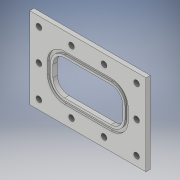
# Autodesk Inventor part: Front
Saved by Autodesk Inventor 2018.1 (Build 221171000, 171)
## iProperties
Created: 2018-04-18
Part Number: Front
Material: Generic
Document SubType Name: Modeling
Designer: trent
Density: 1 g/cm^3
Appearance: Default
Author: trent
Autodesk Inventor part; units mm, degrees
ref_plane "YZ Plane" through (0, 0, 0) normal (1, 0, 0) x (0, 1, 0)
ref_plane "XZ Plane" through (0, 0, 0) normal (0, 1, 0) x (-1, 0, 0)
ref_plane "XY Plane" through (0, 0, 0) normal (0, 0, 1) x (1, 0, 0)
sketch "Sketch1" plane through (0, 0, 0) normal (0, 0, 1) x (1, 0, 0)
  line L0 (0, 0) -> (127, 0)
  line L1 (127, 0) -> (127, 88.9)
  line L2 (127, 88.9) -> (0, 88.9)
  line L3 (0, 88.9) -> (0, 0)
  circle A0 centre (10.16, 78.74) radius 3.0988
  circle A1 centre (10.16, 44.45) radius 3.0988
  circle A2 centre (10.16, 10.16) radius 3.0988
  circle A3 centre (45.72, 10.16) radius 3.0988
  circle A4 centre (116.84, 10.16) radius 3.0988
  circle A5 centre (116.84, 44.45) radius 3.0988
  circle A6 centre (116.84, 78.74) radius 3.0988
  circle A7 centre (45.72, 78.74) radius 3.0988
  line L4 (25.4, 25.4) -> (101.6, 25.4)
  line L5 (101.6, 25.4) -> (101.6, 63.5)
  line L6 (101.6, 63.5) -> (25.4, 63.5)
  line L7 (25.4, 63.5) -> (25.4, 25.4)
  line L8 (25.4, 25.4) -> (101.6, 63.5) construction
  line L9 (101.6, 25.4) -> (25.4, 63.5) construction
  circle A8 centre (81.28, 10.16) radius 3.0988
  circle A9 centre (81.28, 78.74) radius 3.0988
  point P0 (63.5, 44.45)
  dimension "d0" = 127
  dimension "d1" = 88.9
  dimension "d3" = 6.1976
  dimension "d4" = 10.16
  dimension "d5" = 10.16
  dimension "d6" = 10.16
  dimension "d7" = 10.16
  dimension "d8" = 44.45
  dimension "d10" = 10.16
  dimension "d11" = 10.16
  dimension "d12" = 10.16
  dimension "d13" = 10.16
  dimension "d14" = 44.45
  dimension "d15" = 10.16
  dimension "d16" = 10.16
  dimension "d17" = 10.16
  dimension "d18" = 10.16
  dimension "d31" = 76.2
  dimension "d32" = 38.1
  dimension "d33" = 44.45
  dimension "d34" = 63.5
  dimension "d42" = 35.56
  dimension "d43" = 35.56
  dimension "d44" = 35.56
  dimension "d46" = 35.56
  dimension "d47" = 35.56
  dimension "d49" = 35.56
  constraints: 20 end point, 10 centre point, 9 equal radius, 4 parallel, 2 horizontal, 2 midpoint, 2 perpendicular
  measures "d0" distance of L2.end L1.end
  measures "d1" distance of L1.end L0.end
  measures "d3" diameter of A0
  measures "d4" distance from line of L2 A0.centre
  measures "d5" distance from line of L3 A0.centre
  measures "d6" distance from line of L3 A2.centre
  measures "d7" distance from line of L0 A2.centre
  measures "d8" distance from line of L0 A1.centre
  measures "d10" distance from line of L2 A7.centre
  measures "d11" distance from line of L3 A1.centre
  measures "d12" distance from line of L2 A6.centre
  measures "d13" distance from line of L1 A6.centre
  measures "d14" distance from line of L0 A5.centre
  measures "d15" distance from line of L1 A5.centre
  measures "d16" distance from line of L0 A4.centre
  measures "d17" distance from line of L1 A4.centre
  measures "d18" distance from line of L0 A3.centre
  measures "d31" distance of L6.end L5.end
  measures "d32" distance of L5.end L4.end
  measures "d33" distance from line of L0 point (63.5, 44.45)
  measures "d34" distance from line of L1 point (63.5, 44.45)
  measures "d42" distance of A0.centre A7.centre
  measures "d43" distance of A7.centre A9.centre
  measures "d44" distance of A6.centre A9.centre
  measures "d46" distance of A8.centre A3.centre
  measures "d47" distance of A2.centre A3.centre
  measures "d49" distance of A4.centre A8.centre
extrude "Extrusion1" add sketch "Sketch1" along normal blind 4.7625
thread "Thread1" size "M6x1" class "6H" standard "ANSI Metric M Profile" full length
thread "Thread2" size "M6x1" class "6H" standard "ANSI Metric M Profile" full length
thread "Thread3" size "M6x1" class "6H" standard "ANSI Metric M Profile" full length
thread "Thread4" size "M6x1" class "6H" standard "ANSI Metric M Profile" full length
thread "Thread5" size "M6x1" class "6H" standard "ANSI Metric M Profile" full length
thread "Thread6" size "M6x1" class "6H" standard "ANSI Metric M Profile" full length
thread "Thread7" size "M6x1" class "6H" standard "ANSI Metric M Profile" full length
thread "Thread8" size "M6x1" class "6H" standard "ANSI Metric M Profile" full length
thread "Thread9" size "M6x1" class "6H" standard "ANSI Metric M Profile" full length
fillet "Fillet3" radius 12.7 4 edges at (101.6, 63.5, 2.3813) (101.6, 25.4, 2.3813) (25.4, 63.5, 2.3813) (25.4, 25.4, 2.3813)
sketch "Sketch4" plane through (0, 0, 4.7625) normal (0, 0, 1) x (1, 0, 0)
  arc A0 (38.1, 63.5) -> (25.4, 50.8) centre (38.1, 50.8) ccw projected
  arc A1 (38.1, 63.5) -> (25.4, 50.8) centre (38.1, 50.8) ccw
  arc A2 (101.6, 50.8) -> (88.9, 63.5) centre (88.9, 50.8) ccw projected
  arc A3 (101.6, 50.8) -> (88.9, 63.5) centre (88.9, 50.8) ccw
  arc A4 (88.9, 25.4) -> (101.6, 38.1) centre (88.9, 38.1) ccw projected
  arc A5 (88.9, 25.4) -> (101.6, 38.1) centre (88.9, 38.1) ccw
  arc A6 (25.4, 38.1) -> (38.1, 25.4) centre (38.1, 38.1) ccw projected
  arc A7 (25.4, 38.1) -> (38.1, 25.4) centre (38.1, 38.1) ccw
  line L0 (38.1, 25.4) -> (88.9, 25.4) projected
  line L1 (38.1, 25.4) -> (88.9, 25.4)
  line L2 (101.6, 38.1) -> (101.6, 50.8) projected
  line L3 (101.6, 38.1) -> (101.6, 50.8)
  line L4 (88.9, 63.5) -> (38.1, 63.5) projected
  line L5 (88.9, 63.5) -> (38.1, 63.5)
  line L6 (25.4, 38.1) -> (25.4, 50.8) projected
  line L7 (25.4, 50.8) -> (25.4, 38.1)
  arc A8 (38.1, 66.04) -> (22.86, 50.8) centre (38.1, 50.8) ccw
  line L8 (22.86, 50.8) -> (22.86, 38.1)
  arc A9 (22.86, 38.1) -> (38.1, 22.86) centre (38.1, 38.1) ccw
  line L9 (38.1, 22.86) -> (88.9, 22.86)
  arc A10 (88.9, 22.86) -> (104.14, 38.1) centre (88.9, 38.1) ccw
  line L10 (104.14, 38.1) -> (104.14, 50.8)
  arc A11 (104.14, 50.8) -> (88.9, 66.04) centre (88.9, 50.8) ccw
  line L11 (88.9, 66.04) -> (38.1, 66.04)
  arc A12 (38.1, 69.5198) -> (19.3802, 50.8) centre (38.1, 50.8) ccw
  line L12 (19.3802, 50.8) -> (19.3802, 38.1)
  arc A13 (19.3802, 38.1) -> (38.1, 19.3802) centre (38.1, 38.1) ccw
  line L13 (38.1, 19.3802) -> (88.9, 19.3802)
  arc A14 (88.9, 19.3802) -> (107.6198, 38.1) centre (88.9, 38.1) ccw
  line L14 (107.6198, 38.1) -> (107.6198, 50.8)
  arc A15 (107.6198, 50.8) -> (88.9, 69.5198) centre (88.9, 50.8) ccw
  line L15 (88.9, 69.5198) -> (38.1, 69.5198)
  point P0 (0, 0)
  dimension "d69" = 2.54
  dimension "d70" = 3.4798
  constraints: 25 point on circle, 24 end point, 12 centre point, 5 point on line, 4 coincident, 4 tangent, 2 collinear, 1 horizontal, 14 other
  measures "d69" distance between parallel lines of L4 L11
  measures "d70" distance between parallel lines of L11 L15
extrude "Extrusion4" cut sketch "Sketch4" against normal blind 1.9812 contours L15 A15 L14 A14 L13 A13 L12 A12
thread "Thread10" size "M6x1" class "6H" standard "ANSI Metric M Profile" full length
equation "\"d6\" = d5"
equation "\"d7\" = d4"
equation "\"d8\" = 0.5 * d1"
equation "\"d10\" = d4"
equation "\"d11\" = d5"
equation "\"d12\" = d4"
equation "\"d13\" = d5"
equation "\"d14\" = 0.5 * d1"
equation "\"d15\" = d13"
equation "\"d16\" = d12"
equation "\"d17\" = d13"
equation "\"d18\" = d16"
equation "\"d33\" = 0.5 * d1"
equation "\"d34\" = 0.5 * d0"
equation "\"d43\" = d42"
equation "\"d44\" = d43"
equation "\"d46\" = d42"
equation "\"d47\" = d46"
equation "\"d49\" = d46"
body "Solid1"
